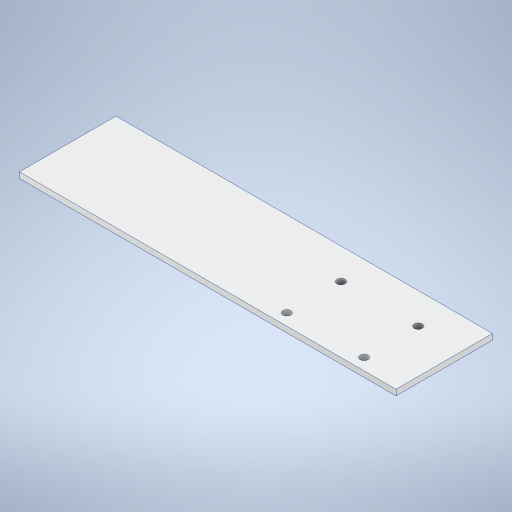
# Autodesk Inventor part: P408
Saved by Autodesk Inventor 2023 (Build 270158000, 158)
## iProperties
Created: 2022-08-30
Part Number: P408
Material: Aluminum 6061
Document SubType Name: Modeling
Designer: D.C. Eksteen
Density: 2.7 g/cm^3
Appearance: Aluminum - Flat
Author: D.C. Eksteen
Title: MOTOR MOUNT PLATE
Autodesk Inventor part; units mm, degrees
ref_plane "YZ Plane" through (0, 0, 0) normal (1, 0, 0) x (0, 1, 0)
ref_plane "XZ Plane" through (0, 0, 0) normal (0, 1, 0) x (-1, 0, 0)
ref_plane "XY Plane" through (0, 0, 0) normal (0, 0, 1) x (1, 0, 0)
sketch "Sketch1" plane through (0, 0, 0) normal (1, 0, 0) x (0, 1, 0)
  line L0 (0, 0) -> (3, 0)
  line L1 (3, 0) -> (3, -50)
  line L2 (3, -50) -> (0, -50)
  line L3 (0, -50) -> (0, 0)
  dimension "d0" = 3
  dimension "d1" = 50
  constraints: 8 end point, 2 parallel, 1 horizontal, 1 perpendicular
  measures "d0" distance of L1.end L2.end
  measures "d1" distance of L0.end L1.end
extrude "Extrusion1" add sketch "Sketch1" along normal blind 195
sketch "Sketch2" plane through (0, 0, -50) normal (0, -1, 0) x (1, 0, 0)
  line L0 (170, 11.4) -> (170, 52.4) projected
  line L1 (175, 52.4) -> (175, 11.4) projected
  arc A0 (170, 11.4) -> (175, 11.4) centre (172.5, 11.4) ccw projected
  arc A1 (175, 52.4) -> (170, 52.4) centre (172.5, 52.4) ccw projected
  line L2 (130, 11.4) -> (130, 52.4) projected
  arc A2 (135, 52.4) -> (130, 52.4) centre (132.5, 52.4) ccw projected
  line L3 (135, 52.4) -> (135, 11.4) projected
  arc A3 (130, 11.4) -> (135, 11.4) centre (132.5, 11.4) ccw projected
  line L4 (170, 11.4) -> (170, 52.4) projected
  arc A4 (175, 52.4) -> (170, 52.4) centre (172.5, 52.4) ccw projected
  line L5 (175, 52.4) -> (175, 11.4) projected
  arc A5 (170, 11.4) -> (175, 11.4) centre (172.5, 11.4) ccw projected
  line L6 (125.45, 0.9) -> (120.45, 5.9) projected
  line L7 (179.55, 0.9) -> (125.45, 0.9) projected
  line L8 (184.55, 5.9) -> (179.55, 0.9) projected
  line L9 (184.55, 52.9) -> (184.55, 5.9) projected
  line L10 (184.55, 52.9) -> (181.55, 52.9) projected
  line L11 (181.55, 52.9) -> (181.55, 64.9) projected
  line L12 (181.55, 64.9) -> (184.55, 64.9) projected
  line L13 (184.55, 65.9) -> (184.55, 64.9) projected
  line L14 (120.45, 65.9) -> (184.55, 65.9) projected
  line L15 (120.45, 65.9) -> (120.45, 64.9) projected
  line L16 (120.45, 64.9) -> (123.45, 64.9) projected
  line L17 (123.45, 64.9) -> (123.45, 52.9) projected
  line L18 (123.45, 52.9) -> (120.45, 52.9) projected
  line L19 (120.45, 52.9) -> (120.45, 5.9) projected
  line L20 (195, 50) -> (195, 0) projected
  line L21 (0, 0) -> (195, 0) projected
  point P0 (0, 50)
  point P1 (132.5, 16)
  point P2 (132.5, 44)
  point P3 (172.5, 16)
  point P4 (172.5, 44)
  dimension "d4" = 22.5
  dimension "d5" = 28
  dimension "d6" = 16
  dimension "d7" = 40
  constraints: 2 horizontal alignment, 2 vertical alignment
  measures "d4" distance from line of L20 point (172.5, 16)
  measures "d5" distance of point (172.5, 16) point (172.5, 44)
  measures "d6" distance from line of L21 point (172.5, 16)
  measures "d7" distance of point (172.5, 44) point (132.5, 44)
hole "Hole1" at (132.5, 0, -34) at (132.5, 0, -6) at (172.5, 0, -34) at (172.5, 0, -6) direction (0, 1, 0) diameter 4 depth 5
body "Solid1"
